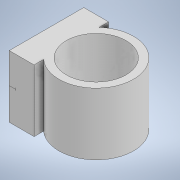
# Autodesk Inventor part: motor mount
Saved by Autodesk Inventor 2022 (Build 260153000, 153)
## iProperties
Created: 2021-07-29
Part Number: motor mount
Material: Generic
Document SubType Name: Modeling
Designer: WASHINGTON
Density: 1 g/cm^3
Appearance: Default
Author: WASHINGTON
Autodesk Inventor part; units mm, degrees
ref_plane "YZ Plane" through (0, 0, 0) normal (1, 0, 0) x (0, 1, 0)
ref_plane "XZ Plane" through (0, 0, 0) normal (0, 1, 0) x (-1, 0, 0)
ref_plane "XY Plane" through (0, 0, 0) normal (0, 0, 1) x (1, 0, 0)
sketch "Sketch1" plane through (0, 0, 0) normal (0, 1, 0) x (-1, 0, 0)
  arc A0 (12, 9) -> (10, -11.1803) centre (0, 0) ccw
  line L0 (10, 15) -> (20, 15)
  line L1 (20, 15) -> (20, -15)
  line L2 (20, -15) -> (10, -15)
  line L3 (10, 15) -> (20, -15) construction
  line L4 (20, 15) -> (10, -15) construction
  line L5 (10, -15) -> (10, -11.1803)
  line L6 (10, 11.1803) -> (10, 15)
  circle A1 centre (0, 0) radius 12
  dimension "d0" = 30
  dimension "d1" = 10
  dimension "d2" = 30
  dimension "d3" = 18.435
  dimension "d4" = 20
  dimension "d5" = 24
  constraints: 14 end point, 3 parallel, 3 point on circle, 2 centre point, 2 coincident, 1 horizontal, 1 perpendicular, 1 point on line, 1 tangent
  measures "d0" diameter of A0
  measures "d1" distance of L1.end L2.end
  measures "d2" distance of L0.end L1.end
  measures "d3" angle of L1 L3
  measures "d4" distance from line of point (0, 0) L1
  measures "d5" diameter of A1
extrude "Extrusion1" add sketch "Sketch1" along normal mid plane 25
sketch "Sketch2" plane through (-20, -12.5, 15) normal (-1, 0, 0) x (0, 0, 1)
  arc A0 (-1.6928, 10.7737) -> (-1.769, 14.7366) centre (-2, 12.75) ccw
  arc A1 (-28.3059, 14.235) -> (-28.2323, 10.2721) centre (-28, 12.2586) ccw
  line L0 (-28.3059, 14.235) -> (-15.5736, 16.2059)
  line L1 (-28.2323, 10.2721) -> (-15.4356, 8.7754)
  line L2 (-14.5668, 16.2249) -> (-1.769, 14.7366)
  line L3 (-14.4239, 8.7945) -> (-1.6928, 10.7737)
  arc A2 (-15.4356, 8.7754) -> (-14.4239, 8.7945) centre (-15, 12.5) ccw
  arc A3 (-14.5668, 16.2249) -> (-15.5736, 16.2059) centre (-15, 12.5) ccw
  dimension "d8" = 4
  dimension "d9" = 4
  dimension "d11" = 26
  dimension "d12" = 13
  constraints: 8 end point, 8 point on circle, 8 tangent, 4 centre point, 1 coincident
  measures "d8" diameter of A1
  measures "d9" diameter of A0
  measures "d11" horizontal distance of A0.centre A1.centre
  measures "d12" horizontal distance of A1.centre point (-15, 12.5)
extrude "Extrusion2" cut sketch "Sketch2" against normal blind 2.5
body "Solid1"
